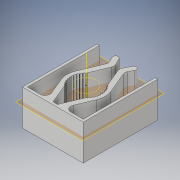
# Autodesk Inventor part: shaft
Saved by Autodesk Inventor 2019.3 (Build 233278000, 278)
## iProperties
Created: 2018-12-19
Part Number: shaft
Material: Generic
Document SubType Name: Modeling
Designer: Frienddo
Density: 1 g/cm^3
Appearance: Default
Author: Frienddo
## iProperties of the stored document shaft toothed clip toothed v2_3DPrint.ipt
Created: 2018-12-20
Part Number: shaft toothed clip toothed v2_3DPrint
Material: Generic
Document SubType Name: Modeling
Designer: Frienddo
Density: 1 g/cm^3
Appearance: Default
Author: Frienddo
Autodesk Inventor part; units mm, degrees
(part 1 of 2)
ref_plane "YZ Plane" through (0, 0, 0) normal (1, 0, 0) x (0, 1, 0)
ref_plane "XZ Plane" through (0, 0, 0) normal (0, 1, 0) x (-1, 0, 0)
ref_plane "XY Plane" through (0, 0, 0) normal (0, 0, 1) x (1, 0, 0)
sketch "Sketch1" plane through (0, 0, 0) normal (0, 1, 0) x (-1, 0, 0)
  line L0 (2.2915, -4.4974) -> (1.9316, -4.6633)
  line L1 (1.9316, -4.6633) -> (1.5598, -4.8005)
  line L2 (1.5598, -4.8005) -> (1.1783, -4.9081)
  line L3 (1.1783, -4.9081) -> (0.7896, -4.9854)
  line L4 (0.7896, -4.9854) -> (0.396, -5.032)
  line L5 (0.396, -5.032) -> (0, -5.0475)
  line L6 (0, -5.0475) -> (-0.396, -5.032)
  line L7 (-0.396, -5.032) -> (-0.7896, -4.9854)
  line L8 (-0.7896, -4.9854) -> (-1.1783, -4.9081)
  line L9 (-1.1783, -4.9081) -> (-1.5598, -4.8005)
  line L10 (-1.5598, -4.8005) -> (-1.9316, -4.6633)
  line L11 (-1.9316, -4.6633) -> (-2.2915, -4.4974)
  line L12 (-2.2915, -4.4974) -> (-2.6373, -4.3037)
  line L13 (-2.6373, -4.3037) -> (-2.9669, -4.0835)
  line L14 (-2.9669, -4.0835) -> (-3.2781, -3.8382)
  line L15 (-3.2781, -3.8382) -> (-3.5692, -3.5692)
  line L16 (-3.5692, -3.5692) -> (-3.8382, -3.2781)
  line L17 (-3.8382, -3.2781) -> (-4.0835, -2.9669)
  line L18 (-4.0835, -2.9669) -> (-4.3037, -2.6373)
  line L19 (-4.3037, -2.6373) -> (-4.4974, -2.2915)
  line L20 (-4.4974, -2.2915) -> (-4.6633, -1.9316)
  line L21 (-4.6633, -1.9316) -> (-4.8005, -1.5598)
  line L22 (-4.8005, -1.5598) -> (-4.9081, -1.1783)
  line L23 (-4.9081, -1.1783) -> (-4.9854, -0.7896)
  line L24 (-4.9854, -0.7896) -> (-5.032, -0.396)
  line L25 (-5.032, -0.396) -> (-5.0475, 0)
  line L26 (-5.0475, 0) -> (-5.032, 0.396)
  line L27 (-5.032, 0.396) -> (-4.9854, 0.7896)
  line L28 (-4.9854, 0.7896) -> (-4.9081, 1.1783)
  line L29 (-4.9081, 1.1783) -> (-4.8005, 1.5598)
  line L30 (-4.8005, 1.5598) -> (-4.6633, 1.9316)
  line L31 (-4.6633, 1.9316) -> (-4.4974, 2.2915)
  line L32 (-4.4974, 2.2915) -> (-4.3037, 2.6373)
  line L33 (-4.3037, 2.6373) -> (-4.0835, 2.9669)
  line L34 (-4.0835, 2.9669) -> (-3.8382, 3.2781)
  line L35 (-3.8382, 3.2781) -> (-3.5692, 3.5692)
  line L36 (-3.5692, 3.5692) -> (-3.2781, 3.8382)
  line L37 (-3.2781, 3.8382) -> (-2.9669, 4.0835)
  line L38 (-2.9669, 4.0835) -> (-2.6373, 4.3037)
  line L39 (-2.6373, 4.3037) -> (-2.2915, 4.4974)
  line L40 (-2.2915, 4.4974) -> (-1.9316, 4.6633)
  line L41 (-1.9316, 4.6633) -> (-1.5598, 4.8005)
  line L42 (-1.5598, 4.8005) -> (-1.1783, 4.9081)
  line L43 (-1.1783, 4.9081) -> (-0.7896, 4.9854)
  line L44 (-0.7896, 4.9854) -> (-0.396, 5.032)
  line L45 (-0.396, 5.032) -> (0, 5.0475)
  line L46 (0, 5.0475) -> (0.396, 5.032)
  line L47 (0.396, 5.032) -> (0.7896, 4.9854)
  line L48 (0.7896, 4.9854) -> (1.1783, 4.9081)
  line L49 (1.1783, 4.9081) -> (1.5598, 4.8005)
  line L50 (1.5598, 4.8005) -> (1.9316, 4.6633)
  line L51 (1.9316, 4.6633) -> (2.2915, 4.4974)
  line L52 (2.2915, 4.4974) -> (2.6373, 4.3037)
  line L53 (2.6373, 4.3037) -> (2.9669, 4.0835)
  line L54 (2.9669, 4.0835) -> (3.2781, 3.8382)
  line L55 (3.2781, 3.8382) -> (3.5692, 3.5692)
  line L56 (3.5692, 3.5692) -> (3.8382, 3.2781)
  line L57 (3.8382, 3.2781) -> (4.0835, 2.9669)
  line L58 (4.0835, 2.9669) -> (4.3037, 2.6373)
  line L59 (4.3037, 2.6373) -> (4.4974, 2.2915)
  line L60 (4.4974, 2.2915) -> (4.6633, 1.9316)
  line L61 (4.6633, 1.9316) -> (4.8005, 1.5598)
  line L62 (4.8005, 1.5598) -> (4.9081, 1.1783)
  line L63 (4.9081, 1.1783) -> (4.9854, 0.7896)
  line L64 (4.9854, 0.7896) -> (5.032, 0.396)
  line L65 (5.032, 0.396) -> (5.0475, 0)
  line L66 (5.0475, 0) -> (5.032, -0.396)
  line L67 (5.032, -0.396) -> (4.9854, -0.7896)
  line L68 (4.9854, -0.7896) -> (4.9081, -1.1783)
  line L69 (4.9081, -1.1783) -> (4.8005, -1.5598)
  line L70 (4.8005, -1.5598) -> (4.6633, -1.9316)
  line L71 (4.6633, -1.9316) -> (4.4974, -2.2915)
  line L72 (4.4974, -2.2915) -> (4.3037, -2.6373)
  line L73 (4.3037, -2.6373) -> (4.0835, -2.9669)
  line L74 (4.0835, -2.9669) -> (3.8382, -3.2781)
  line L75 (3.8382, -3.2781) -> (3.5692, -3.5692)
  line L76 (3.5692, -3.5692) -> (3.2781, -3.8382)
  line L77 (3.2781, -3.8382) -> (2.9669, -4.0835)
  line L78 (2.9669, -4.0835) -> (2.6373, -4.3037)
  line L79 (2.6373, -4.3037) -> (2.2915, -4.4974)
  line L80 (0, 0) -> (0, -5.0475) construction
  circle A0 centre (0, -5.0475) radius 0.25
  circle A1 centre (-0.7896, -4.9854) radius 0.25
  circle A2 centre (-0.4486, -5.7003) radius 0.25
  line L81 (0, -5.0475) -> (-0.4486, -5.7003) construction
  line L82 (-0.4486, -5.7003) -> (-0.7896, -4.9854) construction
  line L83 (-0.4486, -5.7003) -> (0, 0) construction
  line L84 (0.206, -5.1891) -> (-0.2426, -5.8419)
  line L85 (-0.206, -4.9059) -> (-0.6547, -5.5587)
  line L86 (-0.223, -5.5927) -> (-0.564, -4.8778)
  line L87 (-0.6743, -5.8079) -> (-1.0153, -5.093)
  line L88 (0, 0) -> (0.4486, -5.7003) construction
  circle A3 centre (0.4486, -5.7003) radius 0.25
  line L89 (-0.206, -5.1891) -> (0, -5.4889)
  line L90 (0.6547, -5.5587) -> (0.206, -4.9059)
  line L91 (0, -5.0475) -> (0.4486, -5.7003) construction
  line L92 (0, -5.4889) -> (0.2426, -5.8419)
  circle A4 centre (0, 0) radius 3.4236 construction
  circle A5 centre (0, 0) radius 3.4236 construction
  circle A6 centre (1.3348, -5.5599) radius 0.25
  line L93 (0.8587, -5.4213) -> (1.1535, -5.732)
  line L94 (1.5162, -5.3878) -> (0.971, -4.8133)
  line L95 (1.0153, -5.093) -> (0.6743, -5.8079)
  line L96 (0.6083, -5.1575) -> (0.8587, -5.4213)
  circle A7 centre (0.7896, -4.9854) radius 0.25
  line L97 (0.564, -4.8778) -> (0.223, -5.5927)
  circle A8 centre (0.4486, -5.7003) radius 0.25
  circle A9 centre (0, 0) radius 3.4236 construction
  circle A10 centre (2.1882, -5.2827) radius 0.25
  line L98 (1.6962, -5.2203) -> (2.036, -5.481)
  line L99 (2.3403, -5.0843) -> (1.712, -4.6022)
  line L100 (1.7995, -4.8715) -> (1.5745, -5.6309)
  line L101 (1.4076, -4.9988) -> (1.6962, -5.2203)
  circle A11 centre (1.5598, -4.8005) radius 0.25
  line L102 (1.3201, -4.7295) -> (1.0951, -5.4889)
  circle A12 centre (1.3348, -5.5599) radius 0.25
  circle A13 centre (0, 0) radius 3.4236 construction
  circle A14 centre (2.9876, -4.8753) radius 0.25
  line L103 (2.4919, -4.8907) -> (2.8683, -5.095)
  line L104 (3.1069, -4.6556) -> (2.4108, -4.2777)
  line L105 (2.5394, -4.53) -> (2.436, -5.3153)
  line L106 (2.1722, -4.7171) -> (2.4919, -4.8907)
  circle A15 centre (2.2915, -4.4974) radius 0.25
  line L107 (2.0437, -4.4648) -> (1.9403, -5.25)
  circle A16 centre (2.1882, -5.2827) radius 0.25
  circle A17 centre (0, 0) radius 3.4236 construction
  circle A18 centre (3.7135, -4.3479) radius 0.25
  line L108 (3.2263, -4.4406) -> (3.63, -4.5836)
  line L109 (3.7969, -4.1123) -> (3.0503, -3.8479)
  line L110 (3.2168, -4.077) -> (3.2375, -4.8688)
  line L111 (2.8834, -4.3192) -> (3.2263, -4.4406)
  circle A19 centre (2.9669, -4.0835) radius 0.25
  line L112 (2.717, -4.0901) -> (2.7377, -4.8819)
  circle A20 centre (2.9876, -4.8753) radius 0.25
  circle A21 centre (0, 0) radius 3.4236 construction
  circle A22 centre (4.3479, -3.7135) radius 0.25
  line L113 (3.8813, -3.8813) -> (4.3024, -3.9593)
  line L114 (4.3935, -3.4677) -> (3.6147, -3.3233)
  line L115 (3.815, -3.5236) -> (3.9593, -4.3024)
  line L116 (3.5236, -3.815) -> (3.8813, -3.8813)
  circle A23 centre (3.5692, -3.5692) radius 0.25
  line L117 (3.3233, -3.6147) -> (3.4677, -4.3935)
  circle A24 centre (3.7135, -4.3479) radius 0.25
  circle A25 centre (0, 0) radius 3.4236 construction
  circle A26 centre (4.8753, -2.9876) radius 0.25
  line L118 (4.4406, -3.2263) -> (4.8688, -3.2375)
  line L119 (4.8819, -2.7377) -> (4.0901, -2.717)
  line L120 (4.3192, -2.8834) -> (4.5836, -3.63)
  line L121 (4.077, -3.2168) -> (4.4406, -3.2263)
  circle A27 centre (4.0835, -2.9669) radius 0.25
  line L122 (3.8479, -3.0503) -> (4.1123, -3.7969)
  circle A28 centre (4.3479, -3.7135) radius 0.25
  circle A29 centre (0, 0) radius 3.4236 construction
  circle A30 centre (5.2827, -2.1882) radius 0.25
  line L123 (4.8907, -2.4919) -> (5.3153, -2.436)
  line L124 (5.25, -1.9403) -> (4.4648, -2.0437)
  line L125 (4.7171, -2.1722) -> (5.095, -2.8683)
  line L126 (4.53, -2.5394) -> (4.8907, -2.4919)
  circle A31 centre (4.4974, -2.2915) radius 0.25
  line L127 (4.2777, -2.4108) -> (4.6556, -3.1069)
  circle A32 centre (4.8753, -2.9876) radius 0.25
  circle A33 centre (0, 0) radius 3.4236 construction
  circle A34 centre (5.5599, -1.3348) radius 0.25
  line L128 (5.2203, -1.6962) -> (5.6309, -1.5745)
  line L129 (5.4889, -1.0951) -> (4.7295, -1.3201)
  line L130 (4.9988, -1.4076) -> (5.481, -2.036)
  line L131 (4.8715, -1.7995) -> (5.2203, -1.6962)
  circle A35 centre (4.8005, -1.5598) radius 0.25
  line L132 (4.6022, -1.712) -> (5.0843, -2.3403)
  circle A36 centre (5.2827, -2.1882) radius 0.25
  circle A37 centre (0, 0) radius 3.4236 construction
  circle A38 centre (5.7003, -0.4486) radius 0.25
  line L133 (5.4213, -0.8587) -> (5.8079, -0.6743)
  line L134 (5.5927, -0.223) -> (4.8778, -0.564)
  line L135 (5.1575, -0.6083) -> (5.732, -1.1535)
  line L136 (5.093, -1.0153) -> (5.4213, -0.8587)
  circle A39 centre (4.9854, -0.7896) radius 0.25
  line L137 (4.8133, -0.971) -> (5.3878, -1.5162)
  circle A40 centre (5.5599, -1.3348) radius 0.25
  circle A41 centre (0, 0) radius 3.4236 construction
  circle A42 centre (5.7003, 0.4486) radius 0.25
  line L138 (5.4889, 0) -> (5.8419, 0.2426)
  line L139 (5.5587, 0.6547) -> (4.9059, 0.206)
  line L140 (5.1891, 0.206) -> (5.8419, -0.2426)
  line L141 (5.1891, -0.206) -> (5.4889, 0)
  circle A43 centre (5.0475, 0) radius 0.25
  line L142 (4.9059, -0.206) -> (5.5587, -0.6547)
  circle A44 centre (5.7003, -0.4486) radius 0.25
  circle A45 centre (0, 0) radius 3.4236 construction
  circle A46 centre (5.5599, 1.3348) radius 0.25
  line L143 (5.4213, 0.8587) -> (5.732, 1.1535)
  line L144 (5.3878, 1.5162) -> (4.8133, 0.971)
  line L145 (5.093, 1.0153) -> (5.8079, 0.6743)
  line L146 (5.1575, 0.6083) -> (5.4213, 0.8587)
  circle A47 centre (4.9854, 0.7896) radius 0.25
  line L147 (4.8778, 0.564) -> (5.5927, 0.223)
  circle A48 centre (5.7003, 0.4486) radius 0.25
  circle A49 centre (0, 0) radius 3.4236 construction
  circle A50 centre (5.2827, 2.1882) radius 0.25
  line L148 (5.2203, 1.6962) -> (5.481, 2.036)
  line L149 (5.0843, 2.3403) -> (4.6022, 1.712)
  line L150 (4.8715, 1.7995) -> (5.6309, 1.5745)
  line L151 (4.9988, 1.4076) -> (5.2203, 1.6962)
  circle A51 centre (4.8005, 1.5598) radius 0.25
  line L152 (4.7295, 1.3201) -> (5.4889, 1.0951)
  circle A52 centre (5.5599, 1.3348) radius 0.25
  circle A53 centre (0, 0) radius 3.4236 construction
  circle A54 centre (4.8753, 2.9876) radius 0.25
  line L153 (4.8907, 2.4919) -> (5.095, 2.8683)
  line L154 (4.6556, 3.1069) -> (4.2777, 2.4108)
  line L155 (4.53, 2.5394) -> (5.3153, 2.436)
  line L156 (4.7171, 2.1722) -> (4.8907, 2.4919)
  circle A55 centre (4.4974, 2.2915) radius 0.25
  line L157 (4.4648, 2.0437) -> (5.25, 1.9403)
  circle A56 centre (5.2827, 2.1882) radius 0.25
  circle A57 centre (0, 0) radius 3.4236 construction
  circle A58 centre (4.3479, 3.7135) radius 0.25
  line L158 (4.4406, 3.2263) -> (4.5836, 3.63)
  line L159 (4.1123, 3.7969) -> (3.8479, 3.0503)
  line L160 (4.077, 3.2168) -> (4.8688, 3.2375)
  line L161 (4.3192, 2.8834) -> (4.4406, 3.2263)
  circle A59 centre (4.0835, 2.9669) radius 0.25
  line L162 (4.0901, 2.717) -> (4.8819, 2.7377)
  circle A60 centre (4.8753, 2.9876) radius 0.25
  circle A61 centre (0, 0) radius 3.4236 construction
  circle A62 centre (3.7135, 4.3479) radius 0.25
  line L163 (3.8813, 3.8813) -> (3.9593, 4.3024)
  line L164 (3.4677, 4.3935) -> (3.3233, 3.6147)
  line L165 (3.5236, 3.815) -> (4.3024, 3.9593)
  line L166 (3.815, 3.5236) -> (3.8813, 3.8813)
  circle A63 centre (3.5692, 3.5692) radius 0.25
  line L167 (3.6147, 3.3233) -> (4.3935, 3.4677)
  circle A64 centre (4.3479, 3.7135) radius 0.25
  circle A65 centre (0, 0) radius 3.4236 construction
  circle A66 centre (2.9876, 4.8753) radius 0.25
  line L168 (3.2263, 4.4406) -> (3.2375, 4.8688)
  line L169 (2.7377, 4.8819) -> (2.717, 4.0901)
  line L170 (2.8834, 4.3192) -> (3.63, 4.5836)
  line L171 (3.2168, 4.077) -> (3.2263, 4.4406)
  circle A67 centre (2.9669, 4.0835) radius 0.25
  line L172 (3.0503, 3.8479) -> (3.7969, 4.1123)
  circle A68 centre (3.7135, 4.3479) radius 0.25
  circle A69 centre (0, 0) radius 3.4236 construction
  circle A70 centre (2.1882, 5.2827) radius 0.25
  line L173 (2.4919, 4.8907) -> (2.436, 5.3153)
  line L174 (1.9403, 5.25) -> (2.0437, 4.4648)
  line L175 (2.1722, 4.7171) -> (2.8683, 5.095)
  line L176 (2.5394, 4.53) -> (2.4919, 4.8907)
  circle A71 centre (2.2915, 4.4974) radius 0.25
  line L177 (2.4108, 4.2777) -> (3.1069, 4.6556)
  circle A72 centre (2.9876, 4.8753) radius 0.25
  circle A73 centre (0, 0) radius 3.4236 construction
  circle A74 centre (1.3348, 5.5599) radius 0.25
  line L178 (1.6962, 5.2203) -> (1.5745, 5.6309)
  line L179 (1.0951, 5.4889) -> (1.3201, 4.7295)
  line L180 (1.4076, 4.9988) -> (2.036, 5.481)
  line L181 (1.7995, 4.8715) -> (1.6962, 5.2203)
  circle A75 centre (1.5598, 4.8005) radius 0.25
  line L182 (1.712, 4.6022) -> (2.3403, 5.0843)
  circle A76 centre (2.1882, 5.2827) radius 0.25
  circle A77 centre (0, 0) radius 3.4236 construction
  circle A78 centre (0.4486, 5.7003) radius 0.25
  line L183 (0.8587, 5.4213) -> (0.6743, 5.8079)
  line L184 (0.223, 5.5927) -> (0.564, 4.8778)
  line L185 (0.6083, 5.1575) -> (1.1535, 5.732)
  line L186 (1.0153, 5.093) -> (0.8587, 5.4213)
  circle A79 centre (0.7896, 4.9854) radius 0.25
  line L187 (0.971, 4.8133) -> (1.5162, 5.3878)
  circle A80 centre (1.3348, 5.5599) radius 0.25
  circle A81 centre (0, 0) radius 3.4236 construction
  circle A82 centre (-0.4486, 5.7003) radius 0.25
  line L188 (0, 5.4889) -> (-0.2426, 5.8419)
  line L189 (-0.6547, 5.5587) -> (-0.206, 4.9059)
  line L190 (-0.206, 5.1891) -> (0.2426, 5.8419)
  line L191 (0.206, 5.1891) -> (0, 5.4889)
  circle A83 centre (0, 5.0475) radius 0.25
  line L192 (0.206, 4.9059) -> (0.6547, 5.5587)
  circle A84 centre (0.4486, 5.7003) radius 0.25
  circle A85 centre (0, 0) radius 3.4236 construction
  circle A86 centre (-1.3348, 5.5599) radius 0.25
  line L193 (-0.8587, 5.4213) -> (-1.1535, 5.732)
  line L194 (-1.5162, 5.3878) -> (-0.971, 4.8133)
  line L195 (-1.0153, 5.093) -> (-0.6743, 5.8079)
  line L196 (-0.6083, 5.1575) -> (-0.8587, 5.4213)
  circle A87 centre (-0.7896, 4.9854) radius 0.25
  line L197 (-0.564, 4.8778) -> (-0.223, 5.5927)
  circle A88 centre (-0.4486, 5.7003) radius 0.25
  circle A89 centre (0, 0) radius 3.4236 construction
  circle A90 centre (-2.1882, 5.2827) radius 0.25
  line L198 (-1.6962, 5.2203) -> (-2.036, 5.481)
  line L199 (-2.3403, 5.0843) -> (-1.712, 4.6022)
  line L200 (-1.7995, 4.8715) -> (-1.5745, 5.6309)
  line L201 (-1.4076, 4.9988) -> (-1.6962, 5.2203)
  circle A91 centre (-1.5598, 4.8005) radius 0.25
  line L202 (-1.3201, 4.7295) -> (-1.0951, 5.4889)
  circle A92 centre (-1.3348, 5.5599) radius 0.25
  circle A93 centre (0, 0) radius 3.4236 construction
  circle A94 centre (-2.9876, 4.8753) radius 0.25
  line L203 (-2.4919, 4.8907) -> (-2.8683, 5.095)
  line L204 (-3.1069, 4.6556) -> (-2.4108, 4.2777)
  line L205 (-2.5394, 4.53) -> (-2.436, 5.3153)
  line L206 (-2.1722, 4.7171) -> (-2.4919, 4.8907)
  circle A95 centre (-2.2915, 4.4974) radius 0.25
  line L207 (-2.0437, 4.4648) -> (-1.9403, 5.25)
  circle A96 centre (-2.1882, 5.2827) radius 0.25
  circle A97 centre (0, 0) radius 3.4236 construction
  circle A98 centre (-3.7135, 4.3479) radius 0.25
  line L208 (-3.2263, 4.4406) -> (-3.63, 4.5836)
  line L209 (-3.7969, 4.1123) -> (-3.0503, 3.8479)
  line L210 (-3.2168, 4.077) -> (-3.2375, 4.8688)
  line L211 (-2.8834, 4.3192) -> (-3.2263, 4.4406)
  circle A99 centre (-2.9669, 4.0835) radius 0.25
  line L212 (-2.717, 4.0901) -> (-2.7377, 4.8819)
  circle A100 centre (-2.9876, 4.8753) radius 0.25
  circle A101 centre (0, 0) radius 3.4236 construction
  circle A102 centre (-4.3479, 3.7135) radius 0.25
  line L213 (-3.8813, 3.8813) -> (-4.3024, 3.9593)
  line L214 (-4.3935, 3.4677) -> (-3.6147, 3.3233)
  line L215 (-3.815, 3.5236) -> (-3.9593, 4.3024)
  line L216 (-3.5236, 3.815) -> (-3.8813, 3.8813)
  circle A103 centre (-3.5692, 3.5692) radius 0.25
  line L217 (-3.3233, 3.6147) -> (-3.4677, 4.3935)
  circle A104 centre (-3.7135, 4.3479) radius 0.25
  circle A105 centre (0, 0) radius 3.4236 construction
  circle A106 centre (-4.8753, 2.9876) radius 0.25
  line L218 (-4.4406, 3.2263) -> (-4.8688, 3.2375)
  line L219 (-4.8819, 2.7377) -> (-4.0901, 2.717)
  line L220 (-4.3192, 2.8834) -> (-4.5836, 3.63)
  line L221 (-4.077, 3.2168) -> (-4.4406, 3.2263)
  circle A107 centre (-4.0835, 2.9669) radius 0.25
  line L222 (-3.8479, 3.0503) -> (-4.1123, 3.7969)
  circle A108 centre (-4.3479, 3.7135) radius 0.25
  circle A109 centre (0, 0) radius 3.4236 construction
  circle A110 centre (-5.2827, 2.1882) radius 0.25
  line L223 (-4.8907, 2.4919) -> (-5.3153, 2.436)
  line L224 (-5.25, 1.9403) -> (-4.4648, 2.0437)
  line L225 (-4.7171, 2.1722) -> (-5.095, 2.8683)
  line L226 (-4.53, 2.5394) -> (-4.8907, 2.4919)
  circle A111 centre (-4.4974, 2.2915) radius 0.25
  line L227 (-4.2777, 2.4108) -> (-4.6556, 3.1069)
  circle A112 centre (-4.8753, 2.9876) radius 0.25
  circle A113 centre (0, 0) radius 3.4236 construction
  circle A114 centre (-5.5599, 1.3348) radius 0.25
  line L228 (-5.2203, 1.6962) -> (-5.6309, 1.5745)
  line L229 (-5.4889, 1.0951) -> (-4.7295, 1.3201)
  line L230 (-4.9988, 1.4076) -> (-5.481, 2.036)
  line L231 (-4.8715, 1.7995) -> (-5.2203, 1.6962)
  circle A115 centre (-4.8005, 1.5598) radius 0.25
  line L232 (-4.6022, 1.712) -> (-5.0843, 2.3403)
  circle A116 centre (-5.2827, 2.1882) radius 0.25
  circle A117 centre (0, 0) radius 3.4236 construction
  circle A118 centre (-5.7003, 0.4486) radius 0.25
  line L233 (-5.4213, 0.8587) -> (-5.8079, 0.6743)
  line L234 (-5.5927, 0.223) -> (-4.8778, 0.564)
  line L235 (-5.1575, 0.6083) -> (-5.732, 1.1535)
  line L236 (-5.093, 1.0153) -> (-5.4213, 0.8587)
  circle A119 centre (-4.9854, 0.7896) radius 0.25
  line L237 (-4.8133, 0.971) -> (-5.3878, 1.5162)
  circle A120 centre (-5.5599, 1.3348) radius 0.25
  circle A121 centre (0, 0) radius 3.4236 construction
  circle A122 centre (-5.7003, -0.4486) radius 0.25
  line L238 (-5.4889, 0) -> (-5.8419, -0.2426)
  line L239 (-5.5587, -0.6547) -> (-4.9059, -0.206)
  line L240 (-5.1891, -0.206) -> (-5.8419, 0.2426)
  line L241 (-5.1891, 0.206) -> (-5.4889, 0)
  circle A123 centre (-5.0475, 0) radius 0.25
  line L242 (-4.9059, 0.206) -> (-5.5587, 0.6547)
  circle A124 centre (-5.7003, 0.4486) radius 0.25
  circle A125 centre (0, 0) radius 3.4236 construction
  circle A126 centre (-5.5599, -1.3348) radius 0.25
  line L243 (-5.4213, -0.8587) -> (-5.732, -1.1535)
  line L244 (-5.3878, -1.5162) -> (-4.8133, -0.971)
  line L245 (-5.093, -1.0153) -> (-5.8079, -0.6743)
  line L246 (-5.1575, -0.6083) -> (-5.4213, -0.8587)
  circle A127 centre (-4.9854, -0.7896) radius 0.25
  line L247 (-4.8778, -0.564) -> (-5.5927, -0.223)
  circle A128 centre (-5.7003, -0.4486) radius 0.25
  circle A129 centre (0, 0) radius 3.4236 construction
  circle A130 centre (-5.2827, -2.1882) radius 0.25
  line L248 (-5.2203, -1.6962) -> (-5.481, -2.036)
  line L249 (-5.0843, -2.3403) -> (-4.6022, -1.712)
  line L250 (-4.8715, -1.7995) -> (-5.6309, -1.5745)
  line L251 (-4.9988, -1.4076) -> (-5.2203, -1.6962)
  circle A131 centre (-4.8005, -1.5598) radius 0.25
  line L252 (-4.7295, -1.3201) -> (-5.4889, -1.0951)
  circle A132 centre (-5.5599, -1.3348) radius 0.25
  circle A133 centre (0, 0) radius 3.4236 construction
  circle A134 centre (-4.8753, -2.9876) radius 0.25
  line L253 (-4.8907, -2.4919) -> (-5.095, -2.8683)
  line L254 (-4.6556, -3.1069) -> (-4.2777, -2.4108)
  line L255 (-4.53, -2.5394) -> (-5.3153, -2.436)
  line L256 (-4.7171, -2.1722) -> (-4.8907, -2.4919)
  circle A135 centre (-4.4974, -2.2915) radius 0.25
  line L257 (-4.4648, -2.0437) -> (-5.25, -1.9403)
  circle A136 centre (-5.2827, -2.1882) radius 0.25
  circle A137 centre (0, 0) radius 3.4236 construction
  circle A138 centre (-4.3479, -3.7135) radius 0.25
  line L258 (-4.4406, -3.2263) -> (-4.5836, -3.63)
  line L259 (-4.1123, -3.7969) -> (-3.8479, -3.0503)
  line L260 (-4.077, -3.2168) -> (-4.8688, -3.2375)
  line L261 (-4.3192, -2.8834) -> (-4.4406, -3.2263)
  circle A139 centre (-4.0835, -2.9669) radius 0.25
  line L262 (-4.0901, -2.717) -> (-4.8819, -2.7377)
  circle A140 centre (-4.8753, -2.9876) radius 0.25
  circle A141 centre (0, 0) radius 3.4236 construction
  circle A142 centre (-3.7135, -4.3479) radius 0.25
  line L263 (-3.8813, -3.8813) -> (-3.9593, -4.3024)
  line L264 (-3.4677, -4.3935) -> (-3.3233, -3.6147)
  line L265 (-3.5236, -3.815) -> (-4.3024, -3.9593)
  line L266 (-3.815, -3.5236) -> (-3.8813, -3.8813)
  circle A143 centre (-3.5692, -3.5692) radius 0.25
  line L267 (-3.6147, -3.3233) -> (-4.3935, -3.4677)
  circle A144 centre (-4.3479, -3.7135) radius 0.25
  circle A145 centre (0, 0) radius 3.4236 construction
  circle A146 centre (-2.9876, -4.8753) radius 0.25
  line L268 (-3.2263, -4.4406) -> (-3.2375, -4.8688)
  line L269 (-2.7377, -4.8819) -> (-2.717, -4.0901)
  line L270 (-2.8834, -4.3192) -> (-3.63, -4.5836)
  line L271 (-3.2168, -4.077) -> (-3.2263, -4.4406)
  circle A147 centre (-2.9669, -4.0835) radius 0.25
  line L272 (-3.0503, -3.8479) -> (-3.7969, -4.1123)
  circle A148 centre (-3.7135, -4.3479) radius 0.25
  circle A149 centre (0, 0) radius 3.4236 construction
  circle A150 centre (-2.1882, -5.2827) radius 0.25
  line L273 (-2.4919, -4.8907) -> (-2.436, -5.3153)
  line L274 (-1.9403, -5.25) -> (-2.0437, -4.4648)
  line L275 (-2.1722, -4.7171) -> (-2.8683, -5.095)
  line L276 (-2.5394, -4.53) -> (-2.4919, -4.8907)
  circle A151 centre (-2.2915, -4.4974) radius 0.25
  line L277 (-2.4108, -4.2777) -> (-3.1069, -4.6556)
  circle A152 centre (-2.9876, -4.8753) radius 0.25
  circle A153 centre (0, 0) radius 3.4236 construction
  circle A154 centre (-1.3348, -5.5599) radius 0.25
  line L278 (-1.6962, -5.2203) -> (-1.5745, -5.6309)
  line L279 (-1.0951, -5.4889) -> (-1.3201, -4.7295)
  line L280 (-1.4076, -4.9988) -> (-2.036, -5.481)
  line L281 (-1.7995, -4.8715) -> (-1.6962, -5.2203)
  circle A155 centre (-1.5598, -4.8005) radius 0.25
  line L282 (-1.712, -4.6022) -> (-2.3403, -5.0843)
  circle A156 centre (-2.1882, -5.2827) radius 0.25
  circle A157 centre (0, 0) radius 3.4236 construction
  circle A158 centre (-0.4486, -5.7003) radius 0.25
  line L283 (-0.8587, -5.4213) -> (-0.6743, -5.8079)
  line L284 (-0.223, -5.5927) -> (-0.564, -4.8778)
  line L285 (-0.6083, -5.1575) -> (-1.1535, -5.732)
  line L286 (-1.0153, -5.093) -> (-0.8587, -5.4213)
  circle A159 centre (-0.7896, -4.9854) radius 0.25
  line L287 (-0.971, -4.8133) -> (-1.5162, -5.3878)
  circle A160 centre (-1.3348, -5.5599) radius 0.25
  point P0 (0.2426, -5.8419)
  point P1 (0.6547, -5.5587)
  point P2 (1.1535, -5.732)
  point P3 (1.5162, -5.3878)
  point P4 (2.036, -5.481)
  point P5 (2.3403, -5.0843)
  point P6 (2.8683, -5.095)
  point P7 (3.1069, -4.6556)
  point P8 (3.63, -4.5836)
  point P9 (3.7969, -4.1123)
  point P10 (4.3024, -3.9593)
  point P11 (4.3935, -3.4677)
  point P12 (4.8688, -3.2375)
  point P13 (4.8819, -2.7377)
  point P14 (5.3153, -2.436)
  point P15 (5.25, -1.9403)
  point P16 (5.6309, -1.5745)
  point P17 (5.4889, -1.0951)
  point P18 (5.8079, -0.6743)
  point P19 (5.5927, -0.223)
  point P20 (5.8419, 0.2426)
  point P21 (5.5587, 0.6547)
  point P22 (5.732, 1.1535)
  point P23 (5.3878, 1.5162)
  point P24 (5.481, 2.036)
  point P25 (5.0843, 2.3403)
  point P26 (5.095, 2.8683)
  point P27 (4.6556, 3.1069)
  point P28 (4.5836, 3.63)
  point P29 (4.1123, 3.7969)
  point P30 (3.9593, 4.3024)
  point P31 (3.4677, 4.3935)
  point P32 (3.2375, 4.8688)
  point P33 (2.7377, 4.8819)
  point P34 (2.436, 5.3153)
  point P35 (1.9403, 5.25)
  point P36 (1.5745, 5.6309)
  point P37 (1.0951, 5.4889)
  point P38 (0.6743, 5.8079)
  point P39 (0.223, 5.5927)
  point P40 (-0.2426, 5.8419)
  point P41 (-0.6547, 5.5587)
  point P42 (-1.1535, 5.732)
  point P43 (-1.5162, 5.3878)
  point P44 (-2.036, 5.481)
  point P45 (-2.3403, 5.0843)
  point P46 (-2.8683, 5.095)
  point P47 (-3.1069, 4.6556)
  point P48 (-3.63, 4.5836)
  point P49 (-3.7969, 4.1123)
  point P50 (-4.3024, 3.9593)
  point P51 (-4.3935, 3.4677)
  point P52 (-4.8688, 3.2375)
  point P53 (-4.8819, 2.7377)
  point P54 (-5.3153, 2.436)
  point P55 (-5.25, 1.9403)
  point P56 (-5.6309, 1.5745)
  point P57 (-5.4889, 1.0951)
  point P58 (-5.8079, 0.6743)
  point P59 (-5.5927, 0.223)
  point P60 (-5.8419, -0.2426)
  point P61 (-5.5587, -0.6547)
  point P62 (-5.732, -1.1535)
  point P63 (-5.3878, -1.5162)
  point P64 (-5.481, -2.036)
  point P65 (-5.0843, -2.3403)
  point P66 (-5.095, -2.8683)
  point P67 (-4.6556, -3.1069)
  point P68 (-4.5836, -3.63)
  point P69 (-4.1123, -3.7969)
  point P70 (-3.9593, -4.3024)
  point P71 (-3.4677, -4.3935)
  point P72 (-3.2375, -4.8688)
  point P73 (-2.7377, -4.8819)
  point P74 (-2.436, -5.3153)
  point P75 (-1.9403, -5.25)
  point P76 (-1.5745, -5.6309)
  point P77 (-1.0951, -5.4889)
  dimension "d3" = 5.0475
  dimension "d4" = 0.5
  dimension "d5" = 0.5
  dimension "d6" = 0.5
  dimension "d7" = 60
  dimension "d8" = 0.5
  dimension "d9" = 30
  dimension "d12" = 360
  constraints: 576 end point, 402 point on circle, 161 centre point, 42 point on line, 14 tangent, 7 coincident, 1 vertical, 1120 other
  measures "d3" distance of L80.start L5.end
  measures "d4" diameter of A0
  measures "d5" diameter of A1
  measures "d6" diameter of A2
  measures "d7" angle of L82 L81
  measures "d8" diameter of A3
  measures "d9" angle of L88 L91
extrude "Extrusion2" [suppressed]
sketch "Sketch2" plane through (0, 0, 0) normal (0, 1, 0) x (-1, 0, 0)
  line L0 (-0.4094, -5.2018) -> (-0.4961, -5.0201) projected
  line L1 (-0.4961, -5.0201) -> (-0.396, -5.032) projected
  line L2 (-0.396, -5.032) -> (-0.2954, -5.0359) projected
  line L3 (-0.2954, -5.0359) -> (-0.4094, -5.2018) projected
  line L4 (-1.2181, -5.0737) -> (-1.2753, -4.8807) projected
  line L5 (-1.2753, -4.8807) -> (-1.1783, -4.9081) projected
  line L6 (-1.1783, -4.9081) -> (-1.0795, -4.9277) projected
  line L7 (-1.0795, -4.9277) -> (-1.2181, -5.0737) projected
  line L8 (0.4094, -5.2018) -> (0.2954, -5.0359) projected
  line L9 (0.2954, -5.0359) -> (0.396, -5.032) projected
  line L10 (0.396, -5.032) -> (0.4961, -5.0201) projected
  line L11 (0.4961, -5.0201) -> (0.4094, -5.2018) projected
  line L12 (1.2181, -5.0737) -> (1.0795, -4.9277) projected
  line L13 (1.0795, -4.9277) -> (1.1783, -4.9081) projected
  line L14 (1.1783, -4.9081) -> (1.2753, -4.8807) projected
  line L15 (1.2753, -4.8807) -> (1.2181, -5.0737) projected
  line L16 (1.9968, -4.8207) -> (1.8371, -4.6982) projected
  line L17 (1.8371, -4.6982) -> (1.9316, -4.6633) projected
  line L18 (1.9316, -4.6633) -> (2.0231, -4.6212) projected
  line L19 (2.0231, -4.6212) -> (1.9968, -4.8207) projected
  line L20 (2.7264, -4.449) -> (2.5495, -4.353) projected
  line L21 (2.5495, -4.353) -> (2.6373, -4.3037) projected
  line L22 (2.6373, -4.3037) -> (2.7211, -4.2478) projected
  line L23 (2.7211, -4.2478) -> (2.7264, -4.449) projected
  line L24 (3.3888, -3.9677) -> (3.199, -3.9005) projected
  line L25 (3.199, -3.9005) -> (3.2781, -3.8382) projected
  line L26 (3.2781, -3.8382) -> (3.3521, -3.7698) projected
  line L27 (3.3521, -3.7698) -> (3.3888, -3.9677) projected
  line L28 (3.9677, -3.3888) -> (3.7698, -3.3521) projected
  line L29 (3.7698, -3.3521) -> (3.8382, -3.2781) projected
  line L30 (3.8382, -3.2781) -> (3.9005, -3.199) projected
  line L31 (3.9005, -3.199) -> (3.9677, -3.3888) projected
  line L32 (4.449, -2.7264) -> (4.2478, -2.7211) projected
  line L33 (4.2478, -2.7211) -> (4.3037, -2.6373) projected
  line L34 (4.3037, -2.6373) -> (4.353, -2.5495) projected
  line L35 (4.353, -2.5495) -> (4.449, -2.7264) projected
  line L36 (4.8207, -1.9968) -> (4.6212, -2.0231) projected
  line L37 (4.6212, -2.0231) -> (4.6633, -1.9316) projected
  line L38 (4.6633, -1.9316) -> (4.6982, -1.8371) projected
  line L39 (4.6982, -1.8371) -> (4.8207, -1.9968) projected
  line L40 (5.0737, -1.2181) -> (4.8807, -1.2753) projected
  line L41 (4.8807, -1.2753) -> (4.9081, -1.1783) projected
  line L42 (4.9081, -1.1783) -> (4.9277, -1.0795) projected
  line L43 (4.9277, -1.0795) -> (5.0737, -1.2181) projected
  line L44 (5.2018, -0.4094) -> (5.0201, -0.4961) projected
  line L45 (5.0201, -0.4961) -> (5.032, -0.396) projected
  line L46 (5.032, -0.396) -> (5.0359, -0.2954) projected
  line L47 (5.0359, -0.2954) -> (5.2018, -0.4094) projected
  line L48 (5.2018, 0.4094) -> (5.0359, 0.2954) projected
  line L49 (5.0359, 0.2954) -> (5.032, 0.396) projected
  line L50 (5.032, 0.396) -> (5.0201, 0.4961) projected
  line L51 (5.0201, 0.4961) -> (5.2018, 0.4094) projected
  line L52 (5.0737, 1.2181) -> (4.9277, 1.0795) projected
  line L53 (4.9277, 1.0795) -> (4.9081, 1.1783) projected
  line L54 (4.9081, 1.1783) -> (4.8807, 1.2753) projected
  line L55 (4.8807, 1.2753) -> (5.0737, 1.2181) projected
  line L56 (4.8207, 1.9968) -> (4.6982, 1.8371) projected
  line L57 (4.6982, 1.8371) -> (4.6633, 1.9316) projected
  line L58 (4.6633, 1.9316) -> (4.6212, 2.0231) projected
  line L59 (4.6212, 2.0231) -> (4.8207, 1.9968) projected
  line L60 (4.449, 2.7264) -> (4.353, 2.5495) projected
  line L61 (4.353, 2.5495) -> (4.3037, 2.6373) projected
  line L62 (4.3037, 2.6373) -> (4.2478, 2.7211) projected
  line L63 (4.2478, 2.7211) -> (4.449, 2.7264) projected
  line L64 (3.9677, 3.3888) -> (3.9005, 3.199) projected
  line L65 (3.9005, 3.199) -> (3.8382, 3.2781) projected
  line L66 (3.8382, 3.2781) -> (3.7698, 3.3521) projected
  line L67 (3.7698, 3.3521) -> (3.9677, 3.3888) projected
  line L68 (3.3888, 3.9677) -> (3.3521, 3.7698) projected
  line L69 (3.3521, 3.7698) -> (3.2781, 3.8382) projected
  line L70 (3.2781, 3.8382) -> (3.199, 3.9005) projected
  line L71 (3.199, 3.9005) -> (3.3888, 3.9677) projected
  line L72 (2.7264, 4.449) -> (2.7211, 4.2478) projected
  line L73 (2.7211, 4.2478) -> (2.6373, 4.3037) projected
  line L74 (2.6373, 4.3037) -> (2.5495, 4.353) projected
  line L75 (2.5495, 4.353) -> (2.7264, 4.449) projected
  line L76 (1.9968, 4.8207) -> (2.0231, 4.6212) projected
  line L77 (2.0231, 4.6212) -> (1.9316, 4.6633) projected
  line L78 (1.9316, 4.6633) -> (1.8371, 4.6982) projected
  line L79 (1.8371, 4.6982) -> (1.9968, 4.8207) projected
  line L80 (1.2181, 5.0737) -> (1.2753, 4.8807) projected
  line L81 (1.2753, 4.8807) -> (1.1783, 4.9081) projected
  line L82 (1.1783, 4.9081) -> (1.0795, 4.9277) projected
  line L83 (1.0795, 4.9277) -> (1.2181, 5.0737) projected
  line L84 (0.4094, 5.2018) -> (0.4961, 5.0201) projected
  line L85 (0.4961, 5.0201) -> (0.396, 5.032) projected
  line L86 (0.396, 5.032) -> (0.2954, 5.0359) projected
  line L87 (0.2954, 5.0359) -> (0.4094, 5.2018) projected
  line L88 (-0.4094, 5.2018) -> (-0.2954, 5.0359) projected
  line L89 (-0.2954, 5.0359) -> (-0.396, 5.032) projected
  line L90 (-0.396, 5.032) -> (-0.4961, 5.0201) projected
  line L91 (-0.4961, 5.0201) -> (-0.4094, 5.2018) projected
  line L92 (-1.2181, 5.0737) -> (-1.0795, 4.9277) projected
  line L93 (-1.0795, 4.9277) -> (-1.1783, 4.9081) projected
  line L94 (-1.1783, 4.9081) -> (-1.2753, 4.8807) projected
  line L95 (-1.2753, 4.8807) -> (-1.2181, 5.0737) projected
  line L96 (-1.9968, 4.8207) -> (-1.8371, 4.6982) projected
  line L97 (-1.8371, 4.6982) -> (-1.9316, 4.6633) projected
  line L98 (-1.9316, 4.6633) -> (-2.0231, 4.6212) projected
  line L99 (-2.0231, 4.6212) -> (-1.9968, 4.8207) projected
  line L100 (-2.7264, 4.449) -> (-2.5495, 4.353) projected
  line L101 (-2.5495, 4.353) -> (-2.6373, 4.3037) projected
  line L102 (-2.6373, 4.3037) -> (-2.7211, 4.2478) projected
  line L103 (-2.7211, 4.2478) -> (-2.7264, 4.449) projected
  line L104 (-3.3888, 3.9677) -> (-3.199, 3.9005) projected
  line L105 (-3.199, 3.9005) -> (-3.2781, 3.8382) projected
  line L106 (-3.2781, 3.8382) -> (-3.3521, 3.7698) projected
  line L107 (-3.3521, 3.7698) -> (-3.3888, 3.9677) projected
  line L108 (-3.9677, 3.3888) -> (-3.7698, 3.3521) projected
  line L109 (-3.7698, 3.3521) -> (-3.8382, 3.2781) projected
  line L110 (-3.8382, 3.2781) -> (-3.9005, 3.199) projected
  line L111 (-3.9005, 3.199) -> (-3.9677, 3.3888) projected
  line L112 (-4.449, 2.7264) -> (-4.2478, 2.7211) projected
  line L113 (-4.2478, 2.7211) -> (-4.3037, 2.6373) projected
  line L114 (-4.3037, 2.6373) -> (-4.353, 2.5495) projected
  line L115 (-4.353, 2.5495) -> (-4.449, 2.7264) projected
  line L116 (-4.8207, 1.9968) -> (-4.6212, 2.0231) projected
  line L117 (-4.6212, 2.0231) -> (-4.6633, 1.9316) projected
  line L118 (-4.6633, 1.9316) -> (-4.6982, 1.8371) projected
  line L119 (-4.6982, 1.8371) -> (-4.8207, 1.9968) projected
  line L120 (-5.0737, 1.2181) -> (-4.8807, 1.2753) projected
  line L121 (-4.8807, 1.2753) -> (-4.9081, 1.1783) projected
  line L122 (-4.9081, 1.1783) -> (-4.9277, 1.0795) projected
  line L123 (-4.9277, 1.0795) -> (-5.0737, 1.2181) projected
  line L124 (-5.2018, 0.4094) -> (-5.0201, 0.4961) projected
  line L125 (-5.0201, 0.4961) -> (-5.032, 0.396) projected
  line L126 (-5.032, 0.396) -> (-5.0359, 0.2954) projected
  line L127 (-5.0359, 0.2954) -> (-5.2018, 0.4094) projected
  line L128 (-5.2018, -0.4094) -> (-5.0359, -0.2954) projected
  line L129 (-5.0359, -0.2954) -> (-5.032, -0.396) projected
  line L130 (-5.032, -0.396) -> (-5.0201, -0.4961) projected
  line L131 (-5.0201, -0.4961) -> (-5.2018, -0.4094) projected
  line L132 (-5.0737, -1.2181) -> (-4.9277, -1.0795) projected
  line L133 (-4.9277, -1.0795) -> (-4.9081, -1.1783) projected
  line L134 (-4.9081, -1.1783) -> (-4.8807, -1.2753) projected
  line L135 (-4.8807, -1.2753) -> (-5.0737, -1.2181) projected
  line L136 (-4.8207, -1.9968) -> (-4.6982, -1.8371) projected
  line L137 (-4.6982, -1.8371) -> (-4.6633, -1.9316) projected
  line L138 (-4.6633, -1.9316) -> (-4.6212, -2.0231) projected
  line L139 (-4.6212, -2.0231) -> (-4.8207, -1.9968) projected
  line L140 (-4.449, -2.7264) -> (-4.353, -2.5495) projected
  line L141 (-4.353, -2.5495) -> (-4.3037, -2.6373) projected
  line L142 (-4.3037, -2.6373) -> (-4.2478, -2.7211) projected
  line L143 (-4.2478, -2.7211) -> (-4.449, -2.7264) projected
  line L144 (-3.9677, -3.3888) -> (-3.9005, -3.199) projected
  line L145 (-3.9005, -3.199) -> (-3.8382, -3.2781) projected
  line L146 (-3.8382, -3.2781) -> (-3.7698, -3.3521) projected
  line L147 (-3.7698, -3.3521) -> (-3.9677, -3.3888) projected
  line L148 (-3.3888, -3.9677) -> (-3.3521, -3.7698) projected
  line L149 (-3.3521, -3.7698) -> (-3.2781, -3.8382) projected
  line L150 (-3.2781, -3.8382) -> (-3.199, -3.9005) projected
  line L151 (-3.199, -3.9005) -> (-3.3888, -3.9677) projected
  line L152 (-2.7264, -4.449) -> (-2.7211, -4.2478) projected
  line L153 (-2.7211, -4.2478) -> (-2.6373, -4.3037) projected
  line L154 (-2.6373, -4.3037) -> (-2.5495, -4.353) projected
  line L155 (-2.5495, -4.353) -> (-2.7264, -4.449) projected
  line L156 (-1.9968, -4.8207) -> (-2.0231, -4.6212) projected
  line L157 (-2.0231, -4.6212) -> (-1.9316, -4.6633) projected
  line L158 (-1.9316, -4.6633) -> (-1.8371, -4.6982) projected
  line L159 (-1.8371, -4.6982) -> (-1.9968, -4.8207) projected
  arc A0 (-0.6743, -5.8079) -> (-0.2426, -5.8419) centre (-0.4486, -5.7003) ccw projected
  line L160 (-0.2426, -5.8419) -> (0, -5.4889) projected
  line L161 (0, -5.4889) -> (0.2426, -5.8419) projected
  arc A1 (0.2426, -5.8419) -> (0.6743, -5.8079) centre (0.4486, -5.7003) ccw projected
  line L162 (0.6743, -5.8079) -> (0.8587, -5.4213) projected
  line L163 (0.8587, -5.4213) -> (1.1535, -5.732) projected
  arc A2 (1.1535, -5.732) -> (1.5745, -5.6309) centre (1.3348, -5.5599) ccw projected
  line L164 (1.5745, -5.6309) -> (1.6962, -5.2203) projected
  line L165 (1.6962, -5.2203) -> (2.036, -5.481) projected
  arc A3 (2.036, -5.481) -> (2.436, -5.3153) centre (2.1882, -5.2827) ccw projected
  line L166 (2.436, -5.3153) -> (2.4919, -4.8907) projected
  line L167 (2.4919, -4.8907) -> (2.8683, -5.095) projected
  arc A4 (2.8683, -5.095) -> (3.2375, -4.8688) centre (2.9876, -4.8753) ccw projected
  line L168 (3.2375, -4.8688) -> (3.2263, -4.4406) projected
  line L169 (3.2263, -4.4406) -> (3.63, -4.5836) projected
  arc A5 (3.63, -4.5836) -> (3.9593, -4.3024) centre (3.7135, -4.3479) ccw projected
  line L170 (3.9593, -4.3024) -> (3.8813, -3.8813) projected
  line L171 (3.8813, -3.8813) -> (4.3024, -3.9593) projected
  arc A6 (4.3024, -3.9593) -> (4.5836, -3.63) centre (4.3479, -3.7135) ccw projected
  line L172 (4.5836, -3.63) -> (4.4406, -3.2263) projected
  line L173 (4.4406, -3.2263) -> (4.8688, -3.2375) projected
  arc A7 (4.8688, -3.2375) -> (5.095, -2.8683) centre (4.8753, -2.9876) ccw projected
  line L174 (5.095, -2.8683) -> (4.8907, -2.4919) projected
  line L175 (4.8907, -2.4919) -> (5.3153, -2.436) projected
  arc A8 (5.3153, -2.436) -> (5.481, -2.036) centre (5.2827, -2.1882) ccw projected
  line L176 (5.481, -2.036) -> (5.2203, -1.6962) projected
  line L177 (5.2203, -1.6962) -> (5.6309, -1.5745) projected
  arc A9 (5.6309, -1.5745) -> (5.732, -1.1535) centre (5.5599, -1.3348) ccw projected
  line L178 (5.732, -1.1535) -> (5.4213, -0.8587) projected
  line L179 (5.4213, -0.8587) -> (5.8079, -0.6743) projected
  arc A10 (5.8079, -0.6743) -> (5.8419, -0.2426) centre (5.7003, -0.4486) ccw projected
  line L180 (5.8419, -0.2426) -> (5.4889, 0) projected
  line L181 (5.4889, 0) -> (5.8419, 0.2426) projected
  arc A11 (5.8419, 0.2426) -> (5.8079, 0.6743) centre (5.7003, 0.4486) ccw projected
  line L182 (5.8079, 0.6743) -> (5.4213, 0.8587) projected
  line L183 (5.4213, 0.8587) -> (5.732, 1.1535) projected
  arc A12 (5.732, 1.1535) -> (5.6309, 1.5745) centre (5.5599, 1.3348) ccw projected
  line L184 (5.6309, 1.5745) -> (5.2203, 1.6962) projected
  line L185 (5.2203, 1.6962) -> (5.481, 2.036) projected
  arc A13 (5.481, 2.036) -> (5.3153, 2.436) centre (5.2827, 2.1882) ccw projected
  line L186 (5.3153, 2.436) -> (4.8907, 2.4919) projected
  line L187 (4.8907, 2.4919) -> (5.095, 2.8683) projected
  arc A14 (5.095, 2.8683) -> (4.8688, 3.2375) centre (4.8753, 2.9876) ccw projected
  line L188 (4.8688, 3.2375) -> (4.4406, 3.2263) projected
  line L189 (4.4406, 3.2263) -> (4.5836, 3.63) projected
  arc A15 (4.5836, 3.63) -> (4.3024, 3.9593) centre (4.3479, 3.7135) ccw projected
  line L190 (4.3024, 3.9593) -> (3.8813, 3.8813) projected
  line L191 (3.8813, 3.8813) -> (3.9593, 4.3024) projected
  arc A16 (3.9593, 4.3024) -> (3.63, 4.5836) centre (3.7135, 4.3479) ccw projected
  line L192 (3.63, 4.5836) -> (3.2263, 4.4406) projected
  line L193 (3.2263, 4.4406) -> (3.2375, 4.8688) projected
  arc A17 (3.2375, 4.8688) -> (2.8683, 5.095) centre (2.9876, 4.8753) ccw projected
  line L194 (2.8683, 5.095) -> (2.4919, 4.8907) projected
  line L195 (2.4919, 4.8907) -> (2.436, 5.3153) projected
  arc A18 (2.436, 5.3153) -> (2.036, 5.481) centre (2.1882, 5.2827) ccw projected
  line L196 (2.036, 5.481) -> (1.6962, 5.2203) projected
  line L197 (1.6962, 5.2203) -> (1.5745, 5.6309) projected
  arc A19 (1.5745, 5.6309) -> (1.1535, 5.732) centre (1.3348, 5.5599) ccw projected
  line L198 (1.1535, 5.732) -> (0.8587, 5.4213) projected
  line L199 (0.8587, 5.4213) -> (0.6743, 5.8079) projected
  arc A20 (0.6743, 5.8079) -> (0.2426, 5.8419) centre (0.4486, 5.7003) ccw projected
  line L200 (0.2426, 5.8419) -> (0, 5.4889) projected
  line L201 (0, 5.4889) -> (-0.2426, 5.8419) projected
  arc A21 (-0.2426, 5.8419) -> (-0.6743, 5.8079) centre (-0.4486, 5.7003) ccw projected
  line L202 (-0.6743, 5.8079) -> (-0.8587, 5.4213) projected
  line L203 (-0.8587, 5.4213) -> (-1.1535, 5.732) projected
  arc A22 (-1.1535, 5.732) -> (-1.5745, 5.6309) centre (-1.3348, 5.5599) ccw projected
  line L204 (-1.5745, 5.6309) -> (-1.6962, 5.2203) projected
  line L205 (-1.6962, 5.2203) -> (-2.036, 5.481) projected
  arc A23 (-2.036, 5.481) -> (-2.436, 5.3153) centre (-2.1882, 5.2827) ccw projected
  line L206 (-2.436, 5.3153) -> (-2.4919, 4.8907) projected
  line L207 (-2.4919, 4.8907) -> (-2.8683, 5.095) projected
  arc A24 (-2.8683, 5.095) -> (-3.2375, 4.8688) centre (-2.9876, 4.8753) ccw projected
  line L208 (-3.2375, 4.8688) -> (-3.2263, 4.4406) projected
  line L209 (-3.2263, 4.4406) -> (-3.63, 4.5836) projected
  arc A25 (-3.63, 4.5836) -> (-3.9593, 4.3024) centre (-3.7135, 4.3479) ccw projected
  line L210 (-3.9593, 4.3024) -> (-3.8813, 3.8813) projected
  line L211 (-3.8813, 3.8813) -> (-4.3024, 3.9593) projected
  arc A26 (-4.3024, 3.9593) -> (-4.5836, 3.63) centre (-4.3479, 3.7135) ccw projected
  line L212 (-4.5836, 3.63) -> (-4.4406, 3.2263) projected
  line L213 (-4.4406, 3.2263) -> (-4.8688, 3.2375) projected
  arc A27 (-4.8688, 3.2375) -> (-5.095, 2.8683) centre (-4.8753, 2.9876) ccw projected
  line L214 (-5.095, 2.8683) -> (-4.8907, 2.4919) projected
  line L215 (-4.8907, 2.4919) -> (-5.3153, 2.436) projected
  arc A28 (-5.3153, 2.436) -> (-5.481, 2.036) centre (-5.2827, 2.1882) ccw projected
  line L216 (-5.481, 2.036) -> (-5.2203, 1.6962) projected
  line L217 (-5.2203, 1.6962) -> (-5.6309, 1.5745) projected
  arc A29 (-5.6309, 1.5745) -> (-5.732, 1.1535) centre (-5.5599, 1.3348) ccw projected
  line L218 (-5.732, 1.1535) -> (-5.4213, 0.8587) projected
  line L219 (-5.4213, 0.8587) -> (-5.8079, 0.6743) projected
  arc A30 (-5.8079, 0.6743) -> (-5.8419, 0.2426) centre (-5.7003, 0.4486) ccw projected
  line L220 (-5.8419, 0.2426) -> (-5.4889, 0) projected
  line L221 (-5.4889, 0) -> (-5.8419, -0.2426) projected
  arc A31 (-5.8419, -0.2426) -> (-5.8079, -0.6743) centre (-5.7003, -0.4486) ccw projected
  line L222 (-5.8079, -0.6743) -> (-5.4213, -0.8587) projected
  line L223 (-5.4213, -0.8587) -> (-5.732, -1.1535) projected
  arc A32 (-5.732, -1.1535) -> (-5.6309, -1.5745) centre (-5.5599, -1.3348) ccw projected
  line L224 (-5.6309, -1.5745) -> (-5.2203, -1.6962) projected
  line L225 (-5.2203, -1.6962) -> (-5.481, -2.036) projected
  arc A33 (-5.481, -2.036) -> (-5.3153, -2.436) centre (-5.2827, -2.1882) ccw projected
  line L226 (-5.3153, -2.436) -> (-4.8907, -2.4919) projected
  line L227 (-4.8907, -2.4919) -> (-5.095, -2.8683) projected
  arc A34 (-5.095, -2.8683) -> (-4.8688, -3.2375) centre (-4.8753, -2.9876) ccw projected
  line L228 (-4.8688, -3.2375) -> (-4.4406, -3.2263) projected
  line L229 (-4.4406, -3.2263) -> (-4.5836, -3.63) projected
  arc A35 (-4.5836, -3.63) -> (-4.3024, -3.9593) centre (-4.3479, -3.7135) ccw projected
  line L230 (-4.3024, -3.9593) -> (-3.8813, -3.8813) projected
  line L231 (-3.8813, -3.8813) -> (-3.9593, -4.3024) projected
  arc A36 (-3.9593, -4.3024) -> (-3.63, -4.5836) centre (-3.7135, -4.3479) ccw projected
  line L232 (-3.63, -4.5836) -> (-3.2263, -4.4406) projected
  line L233 (-3.2263, -4.4406) -> (-3.2375, -4.8688) projected
  arc A37 (-3.2375, -4.8688) -> (-2.8683, -5.095) centre (-2.9876, -4.8753) ccw projected
  line L234 (-2.8683, -5.095) -> (-2.4919, -4.8907) projected
  line L235 (-2.4919, -4.8907) -> (-2.436, -5.3153) projected
  arc A38 (-2.436, -5.3153) -> (-2.036, -5.481) centre (-2.1882, -5.2827) ccw projected
  line L236 (-2.036, -5.481) -> (-1.6962, -5.2203) projected
  line L237 (-1.6962, -5.2203) -> (-1.5745, -5.6309) projected
  arc A39 (-1.5745, -5.6309) -> (-1.1535, -5.732) centre (-1.3348, -5.5599) ccw projected
  line L238 (-1.1535, -5.732) -> (-0.8587, -5.4213) projected
  line L239 (-0.8587, -5.4213) -> (-0.6743, -5.8079) projected
  line L240 (-3.382, 4.6549) -> (-3.3875, 4.8649)
  arc A40 (-2.7967, 5.2269) -> (-3.3875, 4.8649) centre (-2.9876, 4.8753) ccw
  line L241 (-2.7967, 5.2269) -> (-2.6121, 5.1266)
  line L242 (-2.6121, 5.1266) -> (-2.5847, 5.3349)
  arc A41 (-1.9446, 5.6) -> (-2.5847, 5.3349) centre (-2.1882, 5.2827) ccw
  line L243 (-1.9446, 5.6) -> (-1.778, 5.4721)
  line L244 (-1.778, 5.4721) -> (-1.7184, 5.6735)
  arc A42 (-1.0447, 5.8353) -> (-1.7184, 5.6735) centre (-1.3348, 5.5599) ccw
  line L245 (-1.0447, 5.8353) -> (-0.9001, 5.6829)
  line L246 (-0.9001, 5.6829) -> (-0.8097, 5.8725)
  arc A43 (-0.119, 5.9269) -> (-0.8097, 5.8725) centre (-0.4486, 5.7003) ccw
  line L247 (-0.119, 5.9269) -> (0, 5.7538)
  line L248 (0, 5.7538) -> (0.119, 5.9269)
  arc A44 (0.8097, 5.8725) -> (0.119, 5.9269) centre (0.4486, 5.7003) ccw
  line L249 (0.8097, 5.8725) -> (0.9001, 5.6829)
  line L250 (0.9001, 5.6829) -> (1.0447, 5.8353)
  arc A45 (1.7184, 5.6735) -> (1.0447, 5.8353) centre (1.3348, 5.5599) ccw
  line L251 (1.7184, 5.6735) -> (1.778, 5.4721)
  line L252 (1.778, 5.4721) -> (1.9446, 5.6)
  arc A46 (2.5847, 5.3349) -> (1.9446, 5.6) centre (2.1882, 5.2827) ccw
  line L253 (2.5847, 5.3349) -> (2.6121, 5.1266)
  line L254 (2.6121, 5.1266) -> (2.7967, 5.2269)
  arc A47 (3.3875, 4.8649) -> (2.7967, 5.2269) centre (2.9876, 4.8753) ccw
  line L255 (3.3875, 4.8649) -> (3.382, 4.6549)
  line L256 (3.382, 4.6549) -> (3.58, 4.725)
  arc A48 (4.1068, 4.275) -> (3.58, 4.725) centre (3.7135, 4.3479) ccw
  line L257 (4.1068, 4.275) -> (4.0685, 4.0685)
  line L258 (4.0685, 4.0685) -> (4.275, 4.1068)
  arc A49 (4.725, 3.58) -> (4.275, 4.1068) centre (4.3479, 3.7135) ccw
  line L259 (4.725, 3.58) -> (4.6549, 3.382)
  line L260 (4.6549, 3.382) -> (4.8649, 3.3875)
  arc A50 (5.2269, 2.7967) -> (4.8649, 3.3875) centre (4.8753, 2.9876) ccw
  line L261 (5.2269, 2.7967) -> (5.1266, 2.6121)
  line L262 (5.1266, 2.6121) -> (5.3349, 2.5847)
  arc A51 (5.6, 1.9446) -> (5.3349, 2.5847) centre (5.2827, 2.1882) ccw
  line L263 (5.6, 1.9446) -> (5.4721, 1.778)
  line L264 (5.4721, 1.778) -> (5.6735, 1.7184)
  arc A52 (5.8353, 1.0447) -> (5.6735, 1.7184) centre (5.5599, 1.3348) ccw
  line L265 (5.8353, 1.0447) -> (5.6829, 0.9001)
  line L266 (5.6829, 0.9001) -> (5.8725, 0.8097)
  arc A53 (5.9269, 0.119) -> (5.8725, 0.8097) centre (5.7003, 0.4486) ccw
  line L267 (5.9269, 0.119) -> (5.7538, 0)
  line L268 (5.7538, 0) -> (5.9269, -0.119)
  arc A54 (5.8725, -0.8097) -> (5.9269, -0.119) centre (5.7003, -0.4486) ccw
  line L269 (5.8725, -0.8097) -> (5.6829, -0.9001)
  line L270 (5.6829, -0.9001) -> (5.8353, -1.0447)
  arc A55 (5.6735, -1.7184) -> (5.8353, -1.0447) centre (5.5599, -1.3348) ccw
  line L271 (5.6735, -1.7184) -> (5.4721, -1.778)
  line L272 (5.4721, -1.778) -> (5.6, -1.9446)
  arc A56 (5.3349, -2.5847) -> (5.6, -1.9446) centre (5.2827, -2.1882) ccw
  line L273 (5.3349, -2.5847) -> (5.1266, -2.6121)
  line L274 (5.1266, -2.6121) -> (5.2269, -2.7967)
  arc A57 (4.8649, -3.3875) -> (5.2269, -2.7967) centre (4.8753, -2.9876) ccw
  line L275 (4.8649, -3.3875) -> (4.6549, -3.382)
  line L276 (4.6549, -3.382) -> (4.725, -3.58)
  arc A58 (4.275, -4.1068) -> (4.725, -3.58) centre (4.3479, -3.7135) ccw
  line L277 (4.275, -4.1068) -> (4.0685, -4.0685)
  line L278 (4.0685, -4.0685) -> (4.1068, -4.275)
  arc A59 (3.58, -4.725) -> (4.1068, -4.275) centre (3.7135, -4.3479) ccw
  line L279 (3.58, -4.725) -> (3.382, -4.6549)
  line L280 (3.382, -4.6549) -> (3.3875, -4.8649)
  arc A60 (2.7967, -5.2269) -> (3.3875, -4.8649) centre (2.9876, -4.8753) ccw
  line L281 (2.7967, -5.2269) -> (2.6121, -5.1266)
  line L282 (2.6121, -5.1266) -> (2.5847, -5.3349)
  arc A61 (1.9446, -5.6) -> (2.5847, -5.3349) centre (2.1882, -5.2827) ccw
  line L283 (1.9446, -5.6) -> (1.778, -5.4721)
  line L284 (1.778, -5.4721) -> (1.7184, -5.6735)
  arc A62 (1.0447, -5.8353) -> (1.7184, -5.6735) centre (1.3348, -5.5599) ccw
  line L285 (1.0447, -5.8353) -> (0.9001, -5.6829)
  line L286 (0.9001, -5.6829) -> (0.8097, -5.8725)
  arc A63 (0.119, -5.9269) -> (0.8097, -5.8725) centre (0.4486, -5.7003) ccw
  line L287 (0.119, -5.9269) -> (0, -5.7538)
  line L288 (0, -5.7538) -> (-0.119, -5.9269)
  arc A64 (-0.8097, -5.8725) -> (-0.119, -5.9269) centre (-0.4486, -5.7003) ccw
  line L289 (-0.8097, -5.8725) -> (-0.9001, -5.6829)
  line L290 (-0.9001, -5.6829) -> (-1.0447, -5.8353)
  arc A65 (-1.7184, -5.6735) -> (-1.0447, -5.8353) centre (-1.3348, -5.5599) ccw
  line L291 (-1.7184, -5.6735) -> (-1.778, -5.4721)
  line L292 (-1.778, -5.4721) -> (-1.9446, -5.6)
  arc A66 (-2.5847, -5.3349) -> (-1.9446, -5.6) centre (-2.1882, -5.2827) ccw
  line L293 (-2.5847, -5.3349) -> (-2.6121, -5.1266)
  line L294 (-2.6121, -5.1266) -> (-2.7967, -5.2269)
  arc A67 (-3.3875, -4.8649) -> (-2.7967, -5.2269) centre (-2.9876, -4.8753) ccw
  line L295 (-3.3875, -4.8649) -> (-3.382, -4.6549)
  line L296 (-3.382, -4.6549) -> (-3.58, -4.725)
  arc A68 (-4.1068, -4.275) -> (-3.58, -4.725) centre (-3.7135, -4.3479) ccw
  line L297 (-4.1068, -4.275) -> (-4.0685, -4.0685)
  line L298 (-4.0685, -4.0685) -> (-4.275, -4.1068)
  arc A69 (-4.725, -3.58) -> (-4.275, -4.1068) centre (-4.3479, -3.7135) ccw
  line L299 (-4.725, -3.58) -> (-4.6549, -3.382)
  line L300 (-4.6549, -3.382) -> (-4.8649, -3.3875)
  arc A70 (-5.2269, -2.7967) -> (-4.8649, -3.3875) centre (-4.8753, -2.9876) ccw
  line L301 (-5.2269, -2.7967) -> (-5.1266, -2.6121)
  line L302 (-5.1266, -2.6121) -> (-5.3349, -2.5847)
  arc A71 (-5.6, -1.9446) -> (-5.3349, -2.5847) centre (-5.2827, -2.1882) ccw
  line L303 (-5.6, -1.9446) -> (-5.4721, -1.778)
  line L304 (-5.4721, -1.778) -> (-5.6735, -1.7184)
  arc A72 (-5.8353, -1.0447) -> (-5.6735, -1.7184) centre (-5.5599, -1.3348) ccw
  line L305 (-5.8353, -1.0447) -> (-5.6829, -0.9001)
  line L306 (-5.6829, -0.9001) -> (-5.8725, -0.8097)
  arc A73 (-5.9269, -0.119) -> (-5.8725, -0.8097) centre (-5.7003, -0.4486) ccw
  line L307 (-5.9269, -0.119) -> (-5.7538, 0)
  line L308 (-5.7538, 0) -> (-5.9269, 0.119)
  arc A74 (-5.8725, 0.8097) -> (-5.9269, 0.119) centre (-5.7003, 0.4486) ccw
  line L309 (-5.8725, 0.8097) -> (-5.6829, 0.9001)
  line L310 (-5.6829, 0.9001) -> (-5.8353, 1.0447)
  arc A75 (-5.6735, 1.7184) -> (-5.8353, 1.0447) centre (-5.5599, 1.3348) ccw
  line L311 (-5.6735, 1.7184) -> (-5.4721, 1.778)
  line L312 (-5.4721, 1.778) -> (-5.6, 1.9446)
  arc A76 (-5.3349, 2.5847) -> (-5.6, 1.9446) centre (-5.2827, 2.1882) ccw
  line L313 (-5.3349, 2.5847) -> (-5.1266, 2.6121)
  line L314 (-5.1266, 2.6121) -> (-5.2269, 2.7967)
  arc A77 (-4.8649, 3.3875) -> (-5.2269, 2.7967) centre (-4.8753, 2.9876) ccw
  line L315 (-4.8649, 3.3875) -> (-4.6549, 3.382)
  line L316 (-4.6549, 3.382) -> (-4.725, 3.58)
  arc A78 (-4.275, 4.1068) -> (-4.725, 3.58) centre (-4.3479, 3.7135) ccw
  line L317 (-4.275, 4.1068) -> (-4.0685, 4.0685)
  line L318 (-4.0685, 4.0685) -> (-4.1068, 4.275)
  arc A79 (-3.58, 4.725) -> (-4.1068, 4.275) centre (-3.7135, 4.3479) ccw
  line L319 (-3.58, 4.725) -> (-3.382, 4.6549)
  circle A80 centre (0, 0) radius 7.5
  line L320 (4.0827, 4.5018) -> (0.9109, 12.1152)
  line L321 (6.9232, 2.8843) -> (4.2312, 9.3461)
  line L322 (0.9109, 12.1152) -> (0, 12.1152)
  line L323 (6.0774, 12.1152) -> (11, 12.1152)
  line L324 (11, 12.1152) -> (11, -16.239)
  line L325 (12, 13.1152) -> (0, 13.1152)
  line L326 (12, 13.1152) -> (12, -16.239)
  line L327 (4.0827, -4.5018) -> (1.2313, -11.3461)
  line L328 (6.9232, -2.8843) -> (3.4362, -11.2543)
  line L329 (3.5065, -12.9434) -> (4.4573, -14.7791)
  line L330 (4.0293, -16.127) -> (4.0293, -16.127)
  line L331 (2.6814, -15.699) -> (1.3016, -13.0351)
  arc A81 (6.0774, 12.1152) -> (4.2312, 9.3461) centre (6.0774, 10.1152) ccw
  arc A82 (1.2313, -11.3461) -> (1.3016, -13.0351) centre (3.0775, -12.1152) ccw
  arc A83 (3.4362, -11.2543) -> (3.5065, -12.9434) centre (5.2824, -12.0235) ccw
  arc A84 (4.0293, -16.127) -> (4.4573, -14.7791) centre (3.5694, -15.239) ccw
  arc A85 (2.6814, -15.699) -> (4.0293, -16.127) centre (3.5694, -15.239) ccw
  line L332 (12, -16.239) -> (11, -16.239)
  line L333 (0, -22.3104) -> (0, 19.0195) projected
  line L334 (0, 13.1152) -> (0, 12.1152)
  point P0 (3.0775, 12.1152)
  point P1 (3.0775, -12.1152)
  point P2 (4.9172, -15.667)
  dimension "d16" = 0.15
  dimension "d17" = 15
  dimension "d20" = 130
  dimension "d21" = 2
  dimension "d22" = 2
  dimension "d23" = 10
  dimension "d24" = 10
  dimension "d25" = 2
  dimension "d26" = 4
  dimension "d27" = 2
  dimension "d28" = 1
  dimension "d29" = 1
  dimension "d30" = 1